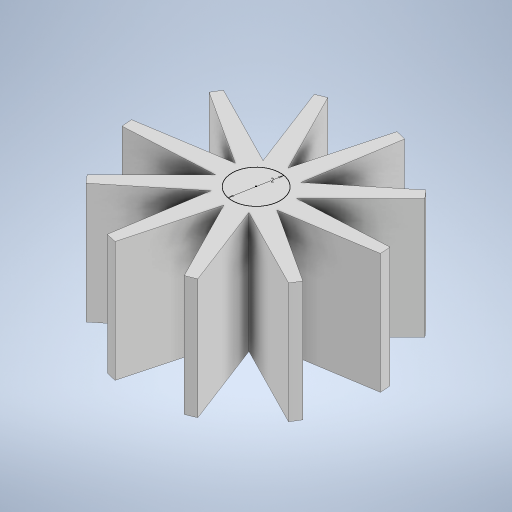
# Autodesk Inventor part: 10ToothGear
Saved by Autodesk Inventor 2024 (Build 280153000, 153)
## iProperties
Created: 2023-07-07
Part Number: 10ToothGear
Material: Generic
Document SubType Name: Modeling
Designer: westy
Density: 1 g/cm^3
Appearance: Default
Author: westy
Autodesk Inventor part; units mm, degrees
ref_plane "YZ Plane" through (0, 0, 0) normal (1, 0, 0) x (0, 1, 0)
ref_plane "XZ Plane" through (0, 0, 0) normal (0, 1, 0) x (-1, 0, 0)
ref_plane "XY Plane" through (0, 0, 0) normal (0, 0, 1) x (1, 0, 0)
sketch "Sketch1" plane through (0, 0, 0) normal (0, 1, 0) x (-1, 0, 0)
  circle A0 centre (0, 0) radius 5
  line L0 (1.7129, -4.6974) -> (0.0019, -1.3369)
  line L1 (0.0019, -1.3369) -> (-0.9539, -4.9082)
  line L2 (4.1469, -2.7935) -> (0.7874, -1.0805)
  line L3 (0.7874, -1.0805) -> (2.1132, -4.5315)
  line L4 (4.9968, 0.1775) -> (1.2721, -0.4113)
  line L5 (1.2721, -0.4113) -> (4.3732, -2.4239)
  line L6 (3.9382, 3.0807) -> (1.2709, 0.4149)
  line L7 (1.2709, 0.4149) -> (4.9627, 0.6095)
  line L8 (1.3753, 4.8071) -> (0.7843, 1.0827)
  line L9 (0.7843, 1.0827) -> (3.6567, 3.4101)
  line L10 (-1.7129, 4.6974) -> (-0.0019, 1.3369)
  line L11 (-0.0019, 1.3369) -> (0.9539, 4.9082)
  line L12 (-4.1469, 2.7935) -> (-0.7874, 1.0805)
  line L13 (-0.7874, 1.0805) -> (-2.1132, 4.5315)
  line L14 (-4.9968, -0.1775) -> (-1.2721, 0.4113)
  line L15 (-1.2721, 0.4113) -> (-4.3732, 2.4239)
  line L16 (-3.9382, -3.0807) -> (-1.2709, -0.4149)
  line L17 (-1.2709, -0.4149) -> (-4.9627, -0.6095)
  line L18 (-1.3753, -4.8071) -> (-0.7843, -1.0827)
  line L19 (-0.7843, -1.0827) -> (-3.6567, -3.4101)
  dimension "d0" = 10
  dimension "d3" = 360
  constraints: 40 end point, 2 point on circle, 1 centre point, 1 coincident, 51 other
  measures "d0" diameter of A0
extrude "Extrusion1" add sketch "Sketch1" along normal blind 5 contours L4 L5 A0 L2 L3 L0 L1 L18 L19 L16 L17 L14 L15 L12 L13 L10 L11 L8 L9 L6 L7
sketch "Sketch2" plane through (0, 5, 0) normal (0, 1, 0) x (1, 0, 0)
  circle A0 centre (0, 0) radius 1
  dimension "d7" = 2
  constraints: 1 centre point, 1 coincident
  measures "d7" diameter of A0
body "Solid1"
